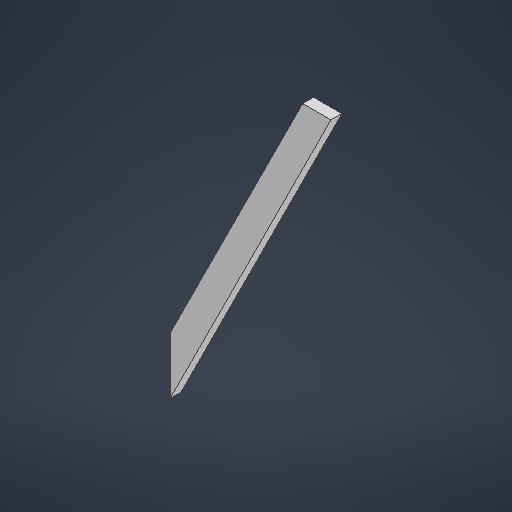
# Autodesk Inventor part: S_2x4x48.13
Saved by Autodesk Inventor 2026 (Build 300175000, 175)
## iProperties
Created: 2025-09-02
Part Number: S_2x4x48.13
Material: Generic
Document SubType Name: Modeling
Designer: trott
Density: 1 g/cm^3
Appearance: Default
Author: trott
Autodesk Inventor part; units mm, degrees
ref_plane "YZ Plane" through (0, 0, 0) normal (1, 0, 0) x (0, 1, 0)
ref_plane "XZ Plane" through (0, 0, 0) normal (0, 1, 0) x (-1, 0, 0)
ref_plane "XY Plane" through (0, 0, 0) normal (0, 0, 1) x (1, 0, 0)
sketch "Sketch1" plane through (0, 0, 0) normal (0, 0, 1) x (1, 0, 0)
  line L0 (0, 0) -> (0, -1219.2)
  line L1 (0, 0) -> (609.6, 0)
  line L2 (0, 0) -> (0, -88.9)
  line L3 (0, -88.9) -> (609.6, -88.9)
  line L4 (609.6, -88.9) -> (609.6, 0)
  line L5 (609.6, 0) -> (0, -1219.2)
  line L6 (565.15, -88.9) -> (485.6354, -49.1427)
  line L7 (485.6354, -49.1427) -> (0, -1020.4136)
  point P0 (0, -1020.4136)
  point P1 (465.7568, -88.9)
  dimension "d0" = 1219.2
  dimension "d1" = 609.6
  dimension "d2" = 88.9
  dimension "d8" = 609.6
  dimension "d9" = 88.9
  dimension "d10" = 90
  constraints: 16 end point, 5 point on line, 2 horizontal, 1 parallel, 1 vertical
  measures "d0" distance of L0.start L0.end
  measures "d1" distance of L0.start L1.end
  measures "d2" distance of L0.start L2.end
  measures "d8" distance of L2.end L3.end
  measures "d9" distance of L6.start L6.end
  measures "d10" angle of L5 L6
extrude "Extrusion1" add sketch "Sketch1" along normal blind 38.1 contours L7 L3 L5 L0
body "Solid1"
